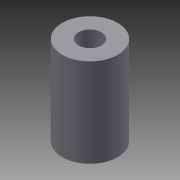
# Autodesk Inventor part: push_clip_rod
Saved by Autodesk Inventor 2015 (Build 190159000, 159)
## iProperties
Created: 2017-10-04
Part Number: push_clip_rod
Material: Generic
Document SubType Name: Modeling
Designer: Anshul
Density: 1 g/cm^3
Appearance: Default
Author: Anshul
Autodesk Inventor part; units mm, degrees
ref_plane "YZ Plane" through (0, 0, 0) normal (1, 0, 0) x (0, 1, 0)
ref_plane "XZ Plane" through (0, 0, 0) normal (0, 1, 0) x (-1, 0, 0)
ref_plane "XY Plane" through (0, 0, 0) normal (0, 0, 1) x (1, 0, 0)
sketch "Sketch1" plane through (0, 0, 0) normal (0, 1, 0) x (-1, 0, 0)
  circle A0 centre (0, 0) radius 1.55
  circle A1 centre (0, 0) radius 3.75
  dimension "d0" = 3.1
  dimension "d1" = 7.5
  constraints: 2 centre point, 2 coincident
  measures "d0" diameter of A0
  measures "d1" diameter of A1
extrude "Extrusion1" add sketch "Sketch1" along normal blind 12
body "Solid1"
